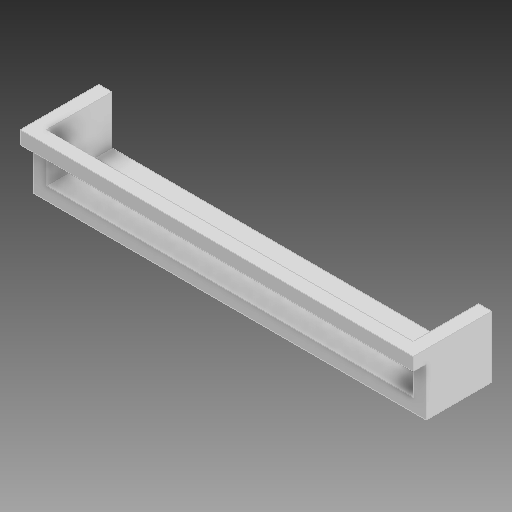
# Autodesk Inventor part: Vorota2
Saved by Autodesk Inventor 2023 (Build 270158000, 158)
## iProperties
Created: 2022-01-19
Part Number: Vorota2
Material: Типовые
Document SubType Name: Modeling
Designer: Администратор
Density: 1 g/cm^3
Appearance: По умолчанию
Author: Администратор
Autodesk Inventor part; units mm, degrees
ref_plane "YZ Plane" through (0, 0, 0) normal (1, 0, 0) x (0, 1, 0)
ref_plane "XZ Plane" through (0, 0, 0) normal (0, 1, 0) x (-1, 0, 0)
ref_plane "XY Plane" through (0, 0, 0) normal (0, 0, 1) x (1, 0, 0)
sketch "Эскиз1" plane through (0, 0, 0) normal (0, 1, 0) x (-1, 0, 0)
  line L0 (-300, 50) -> (300, 50)
  line L1 (300, 50) -> (300, -50)
  line L2 (300, -50) -> (-300, -50)
  line L3 (-300, -50) -> (-300, 50)
  line L4 (0, 50) -> (0, -50) construction
  line L5 (-300, 0) -> (300, 0) construction
  point P0 (0, 0)
  point P1 (0, 0)
  dimension "d0" = 600
  dimension "d1" = 100
  constraints: 12 end point, 5 midpoint, 2 parallel, 1 coincident, 1 horizontal, 1 perpendicular
  measures "d0" distance of L0.start L0.end
  measures "d1" distance of L2.end L0.start
extrude "Выдавливание1" add sketch "Эскиз1" along normal blind 20
sketch "Эскиз2" plane through (0, 20, 0) normal (0, 1, 0) x (1, 0, 0)
  line L0 (300, -50) -> (300, 50) projected
  line L1 (300, 50) -> (-300, 50) projected
  line L2 (300, -50) -> (280, -50)
  line L3 (280, -50) -> (280, 50)
  line L4 (280, 50) -> (300, 50)
  line L5 (300, 50) -> (300, -50)
  line L6 (-300, -50) -> (300, -50) construction
  line L7 (0, -50) -> (0, 50) construction
  line L8 (-300, -50) -> (-300, 50)
  line L9 (-300, -50) -> (-280, -50)
  line L10 (-280, -50) -> (-280, 50)
  line L11 (-280, 50) -> (-300, 50)
  line L12 (-300, 50) -> (-300, -50)
  point P0 (0, 0)
  point P1 (-280, 50)
  dimension "d4" = 20
  constraints: 20 end point, 4 symmetric about line, 2 midpoint, 2 parallel, 1 horizontal, 1 perpendicular, 1 point on line
  measures "d4" distance between parallel lines of L0 L3
extrude "Выдавливание2" add sketch "Эскиз2" along normal blind 74
sketch "Эскиз3" plane through (-300, 0, 50) normal (0, 0, 1) x (1, 0, 0)
  point P0 (300, 0)
sketch "Эскиз4" plane through (0, 0, 0) normal (1, 0, 0) x (0, 1, 0)
  line L0 (20, 50) -> (94, 50) projected
  line L1 (94, 50) -> (74, 50)
  line L2 (74, 50) -> (74, 70)
  line L3 (74, 70) -> (94, 70)
  line L4 (94, 70) -> (94, 50)
  point P0 (0, 0)
  dimension "d7" = 20
  constraints: 8 end point, 2 parallel, 2 perpendicular, 1 horizontal
  measures "d7" distance between parallel lines of L4 L2
extrude "Выдавливание3" add sketch "Эскиз4" along normal mid plane 600
